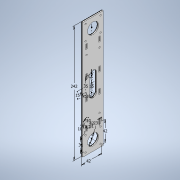
# Autodesk Inventor part: Lateral_Acrilico
Saved by Autodesk Inventor 2021 (Build 250183000, 183)
## iProperties
Created: 2022-08-18
Part Number: Lateral_Acrilico
Material: Genérico
Document SubType Name: Modeling
Designer: 21155060
Density: 1 g/cm^3
Appearance: Padrão
Author: 21155060
Autodesk Inventor part; units mm, degrees
ref_plane "YZ Plane" through (0, 0, 0) normal (1, 0, 0) x (0, 1, 0)
ref_plane "XZ Plane" through (0, 0, 0) normal (0, 1, 0) x (-1, 0, 0)
ref_plane "XY Plane" through (0, 0, 0) normal (0, 0, 1) x (1, 0, 0)
sketch "Esboço1" plane through (0, 0, 0) normal (1, 0, 0) x (0, 1, 0)
  line L0 (-121, -21) -> (121, -21)
  line L1 (121, -21) -> (121, 21)
  line L2 (121, 21) -> (-121, 21)
  line L3 (-121, 21) -> (-121, -21)
  line L4 (-121, -21) -> (121, 21) construction
  line L5 (121, -21) -> (-121, 21) construction
  line L6 (-121, 21) -> (-79, 21) construction
  line L7 (-79, 21) -> (-79, -21) construction
  line L8 (-79, -21) -> (-121, -21) construction
  line L9 (-121, -21) -> (-121, 21) construction
  line L10 (-115.5, -15.5) -> (-84.5, -15.5) construction
  line L11 (-84.5, -15.5) -> (-84.5, 15.5) construction
  line L12 (-84.5, 15.5) -> (-115.5, 15.5) construction
  line L13 (-115.5, 15.5) -> (-115.5, -15.5) construction
  line L14 (-115.5, -15.5) -> (-84.5, 15.5) construction
  line L15 (-84.5, -15.5) -> (-115.5, 15.5) construction
  circle A0 centre (-100, 0) radius 11.5
  line L16 (-25, 0) -> (25, 0) construction
  line L17 (-17.5, -7.5) -> (17.5, -7.5)
  line L18 (17.5, 7.5) -> (-17.5, 7.5)
  arc A1 (-17.5, 7.5) -> (-17.5, -7.5) centre (-17.5, 0) ccw
  arc A2 (17.5, -7.5) -> (17.5, 7.5) centre (17.5, 0) ccw
  line L19 (-79, 15) -> (-68.8, 15)
  line L20 (-68.8, 15) -> (-68.8, 12)
  line L21 (-68.8, 12) -> (-79, 12)
  line L22 (-79, 12) -> (-79, 15)
  line L23 (-25.2, 15) -> (-15, 15)
  line L24 (-15, 15) -> (-15, 12)
  line L25 (-15, 12) -> (-25.2, 12)
  line L26 (-25.2, 12) -> (-25.2, 15)
  circle A3 centre (-58.8, 13.5) radius 5 construction
  line L27 (-121, 0) -> (121, 0) construction
  line L28 (-79, -15) -> (-68.8, -15)
  line L29 (-68.8, -15) -> (-68.8, -12)
  line L30 (-68.8, -12) -> (-79, -12)
  line L31 (-79, -12) -> (-79, -15)
  line L32 (-25.2, -15) -> (-15, -15)
  line L33 (-15, -15) -> (-15, -12)
  line L34 (-15, -12) -> (-25.2, -12)
  line L35 (-25.2, -12) -> (-25.2, -15)
  circle A4 centre (-58.8, -13.5) radius 5 construction
  line L36 (0, -21) -> (0, 21) construction
  circle A5 centre (100, 0) radius 11.5
  line L37 (79, 15) -> (68.8, 15)
  line L38 (68.8, 15) -> (68.8, 12)
  line L39 (68.8, 12) -> (79, 12)
  line L40 (79, 12) -> (79, 15)
  line L41 (25.2, 15) -> (15, 15)
  line L42 (15, 15) -> (15, 12)
  line L43 (15, 12) -> (25.2, 12)
  line L44 (25.2, 12) -> (25.2, 15)
  line L45 (68.8, -15) -> (68.8, -12)
  line L46 (79, -15) -> (68.8, -15)
  line L47 (79, -12) -> (79, -15)
  line L48 (68.8, -12) -> (79, -12)
  line L49 (25.2, -12) -> (25.2, -15)
  line L50 (25.2, -15) -> (15, -15)
  line L51 (15, -12) -> (25.2, -12)
  line L52 (15, -15) -> (15, -12)
  point P0 (0, 0)
  point P1 (-100, 0)
  point P2 (-100, 21)
  point P3 (0, 0)
  point P4 (0, 0)
  point P5 (-68.8, 13.5)
  point P6 (-68.8, -13.5)
  point P7 (68.8, 13.5)
  point P8 (68.8, -13.5)
  dimension "d0" = 242
  dimension "d1" = 42
  dimension "d2" = 42
  dimension "d3" = 42
  dimension "d4" = 31
  dimension "d5" = 31
  dimension "d6" = 23
  dimension "d7" = 15
  dimension "d8" = 35
  dimension "d9" = 10.2
  dimension "d10" = 3
  dimension "d12" = 6
  dimension "d13" = 10.2
  dimension "d14" = 3
  dimension "d15" = 15
  dimension "d16" = 10
  dimension "d17" = 10
  constraints: 108 end point, 29 symmetric about line, 14 midpoint, 11 parallel, 6 centre point, 6 horizontal, 6 point on circle, 5 perpendicular, 4 tangent, 2 coincident, 2 collinear, 2 horizontal alignment, 2 point on line, 1 vertical alignment, 2 other
  measures "d0" distance of L1.end L2.end
  measures "d1" distance of L2.end L0.start
  measures "d2" distance of L7.end L8.end
  measures "d3" distance of L6.end L7.end
  measures "d4" distance of L12.end L11.end
  measures "d5" distance of L11.end L10.end
  measures "d6" diameter of A0
  measures "d7" diameter of A2
  measures "d8" distance of A2.centre A1.centre
  measures "d9" distance of L20.end L21.end
  measures "d10" distance of L19.end L20.end
  measures "d12" distance between parallel lines of L2 L19
  measures "d13" distance of L24.end L25.end
  measures "d14" distance of L23.end L24.end
  measures "d15" distance from line of L24 point (0, 0)
  measures "d16" diameter of A3
  measures "d17" distance from line of L20 A3.centre
extrude "Extrusão1" add sketch "Esboço1" along normal blind 3
hole "Furo1" at (0, -58.8, 13.5) at (0, -58.8, -13.5) at (0, -84.5, 15.5) at (0, -115.5, 15.5) at (0, -115.5, -15.5) at (0, -84.5, -15.5) direction (1, 0, 0) diameter 3 end through all
mirror "Espelhamento1" about plane through (0, 0, 0) normal (0, 1, 0) of "Furo1"
equation "\"d13\" = d9"
equation "\"d14\" = d10"
